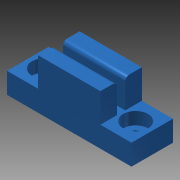
# Autodesk Inventor part: GT2 grip n roll
Saved by Autodesk Inventor 2013 (Build 170138000, 138)
## iProperties
Created: 2017-01-29
Part Number: GT2 grip n roll
Material: Generic
Document SubType Name: Modeling
Designer: Herman de Vries
Density: 1 g/cm^3
Author: Herman de Vries
Autodesk Inventor part; units mm, degrees
ref_plane "YZ Plane" through (0, 0, 0) normal (1, 0, 0) x (0, 1, 0)
ref_plane "XZ Plane" through (0, 0, 0) normal (0, 1, 0) x (-1, 0, 0)
ref_plane "XY Plane" through (0, 0, 0) normal (0, 0, 1) x (1, 0, 0)
sketch "Sketch1" plane through (0, 0, 0) normal (0, 0, 1) x (1, 0, 0)
  line L0 (0, 0) -> (30, 0)
  line L1 (30, 0) -> (30, 10)
  line L2 (30, 10) -> (0, 10)
  line L3 (0, 10) -> (0, 0)
  circle A0 centre (4, 5) radius 1.5
  circle A1 centre (26, 5) radius 1.5
  point P0 (0, 5)
  dimension "d0" = 30
  dimension "d1" = 10
  dimension "d22" = 3
  dimension "d23" = 3
  dimension "d24" = 4
  dimension "d25" = 4
  constraints: 8 end point, 2 centre point, 2 horizontal alignment, 2 parallel, 1 horizontal, 1 midpoint, 1 perpendicular
  measures "d0" distance of L2.end L1.end
  measures "d1" distance of L1.end L0.end
  measures "d22" diameter of A0
  measures "d23" diameter of A1
  measures "d24" distance from line of L3 A0.centre
  measures "d25" distance from line of L1 A1.centre
extrude "Extrusion1" add sketch "Sketch1" along normal blind 5
sketch "Sketch2" plane through (0, 0, 5) normal (0, 0, 1) x (1, 0, 0)
  line L0 (30, 10) -> (0, 10) projected
  line L1 (0, 0) -> (30, 0) projected
  line L2 (7.5, 10) -> (22.5, 10)
  line L3 (22.5, 10) -> (22.5, 6)
  line L4 (22.5, 6) -> (7.5, 6)
  line L5 (7.5, 6) -> (7.5, 10)
  line L6 (7.5, 0) -> (22.5, 0)
  line L7 (22.5, 0) -> (22.5, 4)
  line L8 (22.5, 4) -> (7.5, 4)
  line L9 (7.5, 4) -> (7.5, 0)
  point P0 (15, 10)
  point P1 (15, 10)
  point P2 (15, 0)
  point P3 (15, 0)
  dimension "d14" = 15
  dimension "d15" = 15
  dimension "d31" = 2
  dimension "d32" = 4
  dimension "d33" = 4
  constraints: 16 end point, 4 midpoint, 4 parallel, 2 coincident, 2 horizontal, 2 perpendicular, 2 point on line
  measures "d14" distance of L2.start L2.end
  measures "d15" distance between parallel lines of L9 L7
  measures "d31" distance between parallel lines of L8 L4
  measures "d32" distance of L2.end L3.end
  measures "d33" distance of L6.end L7.end
extrude "Extrusion2" add sketch "Sketch2" along normal blind 7
fillet "Fillet1" radius 1 2 edges at (15, 6, 12) (15, 4, 12)
sketch "Sketch3" plane through (0, 0, 5) normal (0, 0, 1) x (1, 0, 0)
  circle A0 centre (4, 5) radius 1.5 projected
  circle A1 centre (26, 5) radius 1.5 projected
  circle A2 centre (4, 5) radius 3
  circle A3 centre (26, 5) radius 3
  point P0 (0, 0)
  dimension "d35" = 6
  dimension "d36" = 6
  constraints: 2 centre point, 2 coincident
  measures "d35" diameter of A2
  measures "d36" diameter of A3
extrude "Extrusion3" cut sketch "Sketch3" against normal blind 3
equation "\"d15\" = d14"
equation "\"d32\" = d33"
body "Solid1"
